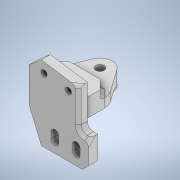
# Autodesk Inventor part: belt_holder_1
Saved by Autodesk Inventor 2020 (Build 240168000, 168)
## iProperties
Created: 2019-05-20
Part Number: belt_holder_1
Material: Generic
Document SubType Name: Modeling
Designer: psrob
Density: 1 g/cm^3
Appearance: Default
Author: psrob
Autodesk Inventor part; units mm, degrees
ref_plane "YZ Plane" through (0, 0, 0) normal (1, 0, 0) x (0, 1, 0)
ref_plane "XZ Plane" through (0, 0, 0) normal (0, 1, 0) x (-1, 0, 0)
ref_plane "XY Plane" through (0, 0, 0) normal (0, 0, 1) x (1, 0, 0)
sketch "Sketch1" plane through (0, 0, 0) normal (0, 0, 1) x (1, 0, 0)
  circle A0 centre (4.591147, -15.25) radius 1.5
  circle A1 centre (11.591147, -15.25) radius 1.5
  circle A2 centre (1.281, 33.75) radius 1
  circle A3 centre (9.281, 32.75) radius 1
  circle A4 centre (-9.854667, 17.759187) radius 1.5
  ellipse E0 centre (11.591147, 1.75) end of major axis (11.591147, 0.25) minor radius 1.5
  ellipse E1 centre (4.591147, 1.75) end of major axis (4.591147, 0.25) minor radius 1.5
  line L0 (15.854667, -21.335738) -> (15.854667, -7.75)
  line L1 (15.854667, -7.75) -> (15.854667, 31.319988)
  arc A5 (15.854667, 31.319988) -> (12.464791, 35.273183) centre (11.854667, 31.319988) ccw
  line L2 (12.464791, 35.273183) -> (-3.583333, 37.75)
  line L3 (-3.583333, 37.75) -> (-15.854667, 37.75)
  line L4 (-15.854667, 37.75) -> (-15.854667, 17.759187)
  arc A6 (-15.854667, 17.759187) -> (-12.464791, 13.805992) centre (-11.854667, 17.759187) ccw
  line L5 (-12.464791, 13.805992) -> (-4.228148, 12.534774)
  arc A7 (0.856667, 6.604982) -> (-4.228148, 12.534774) centre (-5.143333, 6.604982) ccw
  line L6 (0.856667, 6.604982) -> (0.856667, -10.595544)
  arc A8 (-2.560097, -18.122894) -> (0.856667, -10.595544) centre (-9.143333, -10.595544) ccw
  line L7 (-2.560097, -18.122894) -> (-15.854667, -29.75)
  line L8 (-15.854667, -29.75) -> (-15.854667, -37.75)
  line L9 (-15.854667, -37.75) -> (-3.583333, -37.75)
  line L10 (-3.583333, -37.75) -> (13.592861, -22.72812)
  arc A9 (15.854667, -21.335738) -> (13.592861, -22.72812) centre (18.85945, -28.75) ccw
  arc A10 (3.60693, 16.35) -> (6.10693, 16.35) centre (4.85693, 16.35) ccw
  line L11 (3.60693, 16.35) -> (3.60693, 18.35)
  arc A11 (6.10693, 18.35) -> (3.60693, 18.35) centre (4.85693, 18.35) ccw
  line L12 (6.10693, 18.35) -> (6.10693, 16.35)
  arc A12 (10.60934, 16.35) -> (13.10934, 16.35) centre (11.85934, 16.35) ccw
  line L13 (10.60934, 16.35) -> (10.60934, 18.35)
  arc A13 (13.10934, 18.35) -> (10.60934, 18.35) centre (11.85934, 18.35) ccw
  line L14 (13.10934, 18.35) -> (13.10934, 16.35)
  line L15 (-8.583333, 23.75) -> (-8.583333, 27.75)
  arc A14 (-6.583333, 29.75) -> (-8.583333, 27.75) centre (-6.583333, 27.75) ccw
  line L16 (-6.583333, 29.75) -> (9.854667, 29.75)
  arc A15 (11.854667, 27.75) -> (9.854667, 29.75) centre (9.854667, 27.75) ccw
  line L17 (11.854667, 27.75) -> (11.854667, 23.75)
  arc A16 (9.854667, 21.75) -> (11.854667, 23.75) centre (9.854667, 23.75) ccw
  line L18 (9.854667, 21.75) -> (-6.583333, 21.75)
  arc A17 (-8.583333, 23.75) -> (-6.583333, 21.75) centre (-6.583333, 23.75) ccw
  circle A18 centre (-12.719, 33.75) radius 1.5
  circle A19 centre (-6.719, 33.75) radius 1.5
  circle A20 centre (-6.719, -33.75) radius 1.5
  circle A21 centre (-12.719, -33.75) radius 1.5
  circle A22 centre (-9.854667, 17.759187) radius 1.5
  line L19 (-6.228148, 21.534774) -> (-4.228148, 19.534774)
  line L20 (-6.228148, 21.534774) -> (-17.275997, 21.534774)
  ellipse E2 centre (-17.275997, 27.534774) end of major axis (-8.634403, 27.534774) minor radius 6 (-21.607006, 22.342722) -> (-17.275997, 21.534774) ccw
  line L21 (-21.607006, 14.234289) -> (-21.607006, 22.342722)
  ellipse E3 centre (-20.359628, 10.329175) end of major axis (-26.120691, 10.329175) minor radius 4 (-20.359628, 14.329175) -> (-21.607006, 14.234289) ccw
  line L22 (-15.854667, 14.329175) -> (-20.359628, 14.329175)
  line L23 (-15.854667, 14.329175) -> (-7.193044, 12.992367)
  line L24 (-4.228148, 15.534774) -> (-7.193044, 12.992367)
  line L25 (-4.228148, 15.534774) -> (-4.228148, 19.534774)
  line L26 (-3.583333, 37.75) -> (-3.583333, 12.75)
  line L27 (-3.583333, 12.75) -> (15.854667, 12.75)
  line L28 (15.854667, 31.319988) -> (15.854667, 12.75)
  point P0 (0, 0)
  dimension "d0" = 25
  constraints: 6 end point, 1 collinear, 1 perpendicular, 1 point on line, 1 vertical, 2 other
  measures "d0" distance of L2.end L26.end
extrude "Extrusion1" add sketch "Sketch1" along normal blind 4 contours L27 L26 L18 A16 L17 A15 L16 L2 A5 L1 | L26 L16 A15 L17 A16 L18
sketch "Sketch2" plane through (0, 0, 0) normal (0, 0, -1) x (-1, 0, 0)
  line L0 (-9.854667, 29.75) -> (6.583333, 29.75)
  arc A0 (8.583333, 27.75) -> (6.583333, 29.75) centre (6.583333, 27.75) ccw
  line L1 (8.583333, 27.75) -> (8.583333, 23.75)
  circle A1 centre (-1.281, 33.75) radius 1
  circle A2 centre (-9.281, 32.75) radius 1
  circle A3 centre (9.854667, 17.759187) radius 1.5
  ellipse E0 centre (-11.591147, 1.75) end of major axis (-11.591147, 0.25) minor radius 1.5
  ellipse E1 centre (-4.591147, 1.75) end of major axis (-4.591147, 0.25) minor radius 1.5
  arc A4 (-6.10693, 16.35) -> (-3.60693, 16.35) centre (-4.85693, 16.35) ccw
  line L2 (-6.10693, 16.35) -> (-6.10693, 18.35)
  arc A5 (-3.60693, 18.35) -> (-6.10693, 18.35) centre (-4.85693, 18.35) ccw
  line L3 (-3.60693, 18.35) -> (-3.60693, 16.35)
  arc A6 (-13.10934, 16.35) -> (-10.60934, 16.35) centre (-11.85934, 16.35) ccw
  line L4 (-13.10934, 16.35) -> (-13.10934, 18.35)
  arc A7 (-10.60934, 18.35) -> (-13.10934, 18.35) centre (-11.85934, 18.35) ccw
  line L5 (-10.60934, 18.35) -> (-10.60934, 16.35)
  arc A8 (12.464791, 13.805992) -> (15.854667, 17.759187) centre (11.854667, 17.759187) ccw
  line L6 (15.854667, 17.759187) -> (15.854667, 37.75)
  line L7 (3.583333, 37.75) -> (15.854667, 37.75)
  line L8 (3.583333, 37.75) -> (-12.464791, 35.273183)
  arc A9 (-12.464791, 35.273183) -> (-15.854667, 31.319988) centre (-11.854667, 31.319988) ccw
  line L9 (-15.854667, 31.319988) -> (-15.854667, -3.75)
  line L10 (-0.856667, -3.75) -> (-15.854667, -3.75)
  line L11 (-0.856667, 6.604982) -> (-0.856667, -3.75)
  arc A10 (4.228148, 12.534774) -> (-0.856667, 6.604982) centre (5.143333, 6.604982) ccw
  line L12 (4.228148, 12.534774) -> (12.464791, 13.805992)
  circle A11 centre (6.719, 33.75) radius 1.5
  circle A12 centre (12.719, 33.75) radius 1.5
  line L13 (-9.854667, 29.75) -> (6.583333, 29.75)
  arc A13 (8.583333, 27.75) -> (6.583333, 29.75) centre (6.583333, 27.75) ccw
  line L14 (8.583333, 27.75) -> (8.583333, 23.75)
  arc A14 (6.583333, 21.75) -> (8.583333, 23.75) centre (6.583333, 23.75) ccw
  line L15 (6.583333, 21.75) -> (-9.854667, 21.75)
  arc A15 (-11.854667, 23.75) -> (-9.854667, 21.75) centre (-9.854667, 23.75) ccw
  line L16 (-11.854667, 23.75) -> (-11.854667, 27.75)
  arc A16 (-9.854667, 29.75) -> (-11.854667, 27.75) centre (-9.854667, 27.75) ccw
  line L17 (-9.854667, 27.75) -> (6.583333, 23.75)
  line L18 (6.583333, 23.75) -> (6.583333, 27.75)
  line L19 (6.583333, 27.75) -> (-9.854667, 23.75)
  line L20 (-9.635667, 28.25) -> (6.364333, 28.25)
  line L21 (6.364333, 28.25) -> (6.364333, 23.25)
  line L22 (6.364333, 23.25) -> (-9.635667, 23.25)
  line L23 (-9.635667, 23.25) -> (-9.635667, 28.25)
  line L24 (-9.635667, 28.25) -> (6.364333, 23.25) construction
  line L25 (6.364333, 28.25) -> (-9.635667, 23.25) construction
  point P0 (0, 0)
  point P1 (-1.635667, 25.75)
  dimension "d3" = 16
  dimension "d4" = 5
  constraints: 18 end point, 3 midpoint, 2 parallel, 1 horizontal, 1 perpendicular, 1 vertical, 2 other
  measures "d3" distance of L20.start L20.end
  measures "d4" distance of L20.end L21.end
extrude "Extrusion2" add sketch "Sketch2" along normal blind 10 contours L23 L20 L21 L19 L17 | L17 L19 L23 | L19 L21 L17 | L17 L21 L22 L23 L19
sketch "Sketch5" plane through (-6.364333, 28.25, 0) normal (0, 1, 0) x (1, 0, 0)
  line L0 (0, 0) -> (2.781, 0)
  line L1 (16, 0) -> (2.781, 0)
  line L2 (16, 0) -> (16, 10)
  line L3 (0, 10) -> (16, 10)
  line L4 (0, 0) -> (0, 10)
  circle A0 centre (21.963546, 21.566956) radius 5.35
  circle A1 centre (-9.490334, 18.594839) radius 3.75
  circle A2 centre (21.963546, 21.566956) radius 6
  circle A3 centre (-9.490334, 18.594839) radius 6
  line L5 (21.963546, 21.566956) -> (-9.490334, 18.594839)
  line L6 (6.236606, 20.080897) -> (6.42475, 18.089766)
  line L7 (6.42475, 18.089766) -> (1.944706, 17.666441)
  line L8 (1.944706, 17.666441) -> (10.904795, 18.513092)
  circle A4 centre (10.904795, 18.513092) radius 4.5
  circle A5 centre (1.944706, 17.666441) radius 4.5
  circle A6 centre (10.904795, 18.513092) radius 2.5
  circle A7 centre (1.944706, 17.666441) radius 2.5
  line L9 (10.904795, 18.513092) -> (10.669614, 21.002005)
  line L10 (10.669614, 21.002005) -> (1.709526, 20.155355)
  line L11 (1.944706, 17.666441) -> (1.709526, 20.155355)
  line L12 (16, 10) -> (13.393708, 18.748272)
  line L13 (0, 10) -> (-0.548603, 17.483665)
  line L14 (1.944706, 17.666441) -> (-0.548603, 17.483665)
  line L15 (10.904795, 18.513092) -> (13.393708, 18.748272)
  point P0 (6.364333, 0)
  dimension "d15" = 12
  dimension "d16" = 12
  dimension "d17" = 2
  dimension "d18" = 4.5
  dimension "d19" = 9
  dimension "d20" = 9
  dimension "d21" = 9
  dimension "d22" = 5
  dimension "d23" = 5
  constraints: 22 end point, 6 centre point, 6 coincident, 5 perpendicular, 4 point on circle, 3 point on line, 1 midpoint, 1 parallel
  measures "d15" diameter of A2
  measures "d16" diameter of A3
  measures "d17" distance of L6.start L6.end
  measures "d18" distance of L6.end L7.end
  measures "d19" distance of L7.end L8.end
  measures "d20" diameter of A4
  measures "d21" diameter of A5
  measures "d22" diameter of A6
  measures "d23" diameter of A7
extrude "Extrusion5" add sketch "Sketch5" against normal up to surface (5 mm away) contours L13 A5 A4 L12 L3 | L13 A7 L7 A5 | A4 L8 A6 L12 | L14 L7 A7 | A7 L5 L11 L14 | A5 L5 L6 | A4 L5 A6 L8 | L6 L5 A4 | L7 A7 L5 A5 | L15 L9 L5 A6 | A6 L8 L15 | A7 L11 L5 | L10 A4 L5 A5 | A5 L5 A7 L10 | L11 L5 A7 L7 | A6 L5 L9 L8 | A4 L10 A6 L5 | L5 L9 A6 | L11 A7 L5 | A6 L9 L5 picked at (3.816876, 20.111221) picked at (8.607828, 20.563924)
thicken "Thicken1" operation add thickness 1 both sides no extend neighbours yes toward (0, -1, 0) faces at (-0.104, 23.25, -6.666667)
sketch "Sketch6" plane through (-6.364333, 28.25, 0) normal (0, 1, 0) x (1, 0, 0)
  line L0 (0, 0) -> (2.781, 0)
  line L1 (16, 0) -> (2.781, 0)
  line L2 (16, 0) -> (16, 10)
  line L3 (16, 10) -> (13.393708, 18.748272)
  arc A0 (13.393708, 18.748272) -> (10.669614, 21.002005) centre (10.904795, 18.513092) ccw
  line L4 (10.669614, 21.002005) -> (1.709526, 20.155355)
  arc A1 (1.709526, 20.155355) -> (-0.548603, 17.483665) centre (1.944706, 17.666441) ccw
  line L5 (-0.548603, 17.483665) -> (0, 10)
  line L6 (0, 0) -> (0, 10)
  line L7 (10.904795, 18.513092) -> (1.944706, 17.666441)
  line L8 (31.878318, 14.46818) -> (-17.899951, 9.764568)
  line L9 (-17.899951, 9.764568) -> (-19.028817, 21.711353)
  line L10 (-19.028817, 21.711353) -> (30.749451, 26.414965)
  line L11 (30.749451, 26.414965) -> (31.878318, 14.46818)
  line L12 (31.878318, 14.46818) -> (-19.028817, 21.711353) construction
  line L13 (-17.899951, 9.764568) -> (30.749451, 26.414965) construction
  point P0 (6.364333, 0)
  point P1 (6.42475, 18.089766)
  dimension "d28" = 50
  dimension "d29" = 12
  constraints: 14 end point, 3 midpoint, 2 parallel, 1 perpendicular
  measures "d28" distance of L8.start L8.end
  measures "d29" distance of L8.end L9.end
extrude "Extrusion6" cut sketch "Sketch6" against normal blind 3 contours L8 L9 L10 L11 L3 A0 L4 A1 L5 | L5 A1 L4 A0 L3 L8
sketch "Sketch9" plane through (0, 0, 0) normal (0, 0, -1) x (-1, 0, 0)
  line L0 (-9.635667, 28.25) -> (3.583333, 28.25)
  line L1 (3.583333, 37.75) -> (3.583333, 28.25)
  line L2 (-12.464791, 35.273183) -> (3.583333, 37.75)
  arc A0 (-12.464791, 35.273183) -> (-15.854667, 31.319988) centre (-11.854667, 31.319988) ccw
  line L3 (-15.854667, 12.75) -> (-15.854667, 31.319988)
  line L4 (3.583333, 12.75) -> (-15.854667, 12.75)
  line L5 (3.583333, 22.25) -> (3.583333, 12.75)
  line L6 (3.583333, 22.25) -> (-9.635667, 22.25)
  line L7 (-9.635667, 22.25) -> (-9.635667, 28.25)
  circle A1 centre (-1.281, 33.75) radius 1
  circle A2 centre (-9.281, 32.75) radius 1
  arc A3 (-13.10934, 16.35) -> (-10.60934, 16.35) centre (-11.85934, 16.35) ccw
  line L8 (-13.10934, 18.35) -> (-13.10934, 16.35)
  arc A4 (-10.60934, 18.35) -> (-13.10934, 18.35) centre (-11.85934, 18.35) ccw
  line L9 (-10.60934, 16.35) -> (-10.60934, 18.35)
  arc A5 (-6.10693, 16.35) -> (-3.60693, 16.35) centre (-4.85693, 16.35) ccw
  line L10 (-6.10693, 18.35) -> (-6.10693, 16.35)
  arc A6 (-3.60693, 18.35) -> (-6.10693, 18.35) centre (-4.85693, 18.35) ccw
  line L11 (-3.60693, 16.35) -> (-3.60693, 18.35)
  arc A7 (-12.464791, 35.273183) -> (-15.854667, 31.319988) centre (-11.854667, 31.319988) ccw
  line L12 (-15.854667, 12.75) -> (-15.854667, 31.319988)
  line L13 (-12.464791, 35.273183) -> (-15.854667, 35.273183)
  line L14 (-15.854667, 35.273183) -> (-15.854667, 22.25)
  line L15 (-15.854667, 22.25) -> (-12.464791, 22.25)
  line L16 (-12.464791, 22.25) -> (-12.464791, 35.273183)
  point P0 (0, 0)
  point P1 (-15.854667, 31.319988)
  constraints: 8 end point, 2 parallel, 1 horizontal, 1 perpendicular, 1 point on line
extrude "Extrusion9" cut sketch "Sketch9" against normal blind 4 contours L16 L15 L3 A0 | A0 L14 L13
sketch "Sketch10" plane through (0, 0, 0) normal (0, 0, -1) x (-1, 0, 0)
  line L0 (-12.464791, 22.25) -> (-15.854667, 22.25)
  line L1 (-15.854667, 12.75) -> (-15.854667, 22.25)
  line L2 (3.583333, 12.75) -> (-15.854667, 12.75)
  line L3 (3.583333, 22.25) -> (3.583333, 12.75)
  line L4 (3.583333, 22.25) -> (-9.635667, 22.25)
  line L5 (-9.635667, 22.25) -> (-9.635667, 28.25)
  line L6 (-9.635667, 28.25) -> (3.583333, 28.25)
  line L7 (3.583333, 37.75) -> (3.583333, 28.25)
  line L8 (-12.464791, 35.273183) -> (3.583333, 37.75)
  line L9 (-12.464791, 35.273183) -> (-12.464791, 22.25)
  circle A0 centre (-1.281, 33.75) radius 1
  circle A1 centre (-9.281, 32.75) radius 1
  arc A2 (-13.10934, 16.35) -> (-10.60934, 16.35) centre (-11.85934, 16.35) ccw
  line L10 (-13.10934, 18.35) -> (-13.10934, 16.35)
  arc A3 (-10.60934, 18.35) -> (-13.10934, 18.35) centre (-11.85934, 18.35) ccw
  line L11 (-10.60934, 16.35) -> (-10.60934, 18.35)
  arc A4 (-6.10693, 16.35) -> (-3.60693, 16.35) centre (-4.85693, 16.35) ccw
  line L12 (-6.10693, 18.35) -> (-6.10693, 16.35)
  arc A5 (-3.60693, 18.35) -> (-6.10693, 18.35) centre (-4.85693, 18.35) ccw
  line L13 (-3.60693, 16.35) -> (-3.60693, 18.35)
  line L14 (3.583333, 12.75) -> (-15.854667, 12.75)
  line L15 (3.583333, 12.75) -> (-0.416667, 12.75)
  line L16 (-0.416667, 12.75) -> (-0.416667, 22.25)
  line L17 (-0.416667, 22.25) -> (3.583333, 22.25)
  line L18 (3.583333, 22.25) -> (3.583333, 12.75)
  point P0 (0, 0)
  dimension "d44" = 4
  dimension "d45" = 9.5
  constraints: 8 end point, 2 parallel, 1 horizontal, 1 perpendicular
  measures "d44" distance of L16.end L17.end
  measures "d45" distance of L15.end L16.end
extrude "Extrusion10" cut sketch "Sketch10" against normal blind 4 contours L16 L4 L3 L2
sketch "Sketch11" plane through (-6.364333, 22.25, 0) normal (0, -1, 0) x (1, 0, 0)
  line L0 (16, -10) -> (13.393708, -18.748272)
  line L1 (16, 0) -> (16, -10)
  line L2 (6.781, 0) -> (16, 0)
  line L3 (6.781, 0) -> (6.781, 4)
  line L4 (2.781, 4) -> (6.781, 4)
  line L5 (2.781, 0) -> (2.781, 4)
  line L6 (2.781, 0) -> (0, 0)
  line L7 (0, 0) -> (0, -10)
  line L8 (-0.548603, -17.483665) -> (0, -10)
  line L9 (10.669614, -21.002005) -> (1.709526, -20.155355)
  line L10 (0, 0) -> (0, -4)
  line L11 (0, 0) -> (0, -10)
  line L12 (0, -4) -> (2.781, 0)
  arc A0 (-0.548603, -17.483665) -> (1.709526, -20.155355) centre (1.944706, -17.666441) ccw
  arc A1 (10.669614, -21.002005) -> (13.393708, -18.748272) centre (10.904795, -18.513092) ccw
  point P0 (6.364333, 0)
  dimension "d48" = 4
  constraints: 4 end point, 1 point on line
  measures "d48" distance of L6.end L10.end
extrude "Extrusion11" cut sketch "Sketch11" against normal blind 6 contours L12 L7 L6
sketch "Sketch12" plane through (9.635667, 28.25, 0) normal (0, 1, 0) x (1, 0, 0)
  line L0 (-16, 4) -> (-13.219, 0)
  line L1 (0, 0) -> (-13.219, 0)
  line L2 (0, 0) -> (0, 10)
  line L3 (0, 10) -> (-0.859966, 12.886558)
  line L4 (-0.859966, 12.886558) -> (-16.105997, 11.445942)
  line L5 (-16.105997, 11.445942) -> (-16, 10)
  line L6 (-16, 4) -> (-16, 10)
  line L7 (-16.105997, 11.445942) -> (-13.119301, 11.728158)
  line L8 (-0.859966, 12.886558) -> (-16.105997, 11.445942)
  line L9 (-13.119301, 11.728158) -> (-16, 10)
  line L10 (-0.859966, 12.886558) -> (-3.846662, 12.604342)
  line L11 (-3.846662, 12.604342) -> (0, 10)
  point P0 (-9.635667, 0)
  dimension "d51" = 3
  dimension "d52" = 3
  constraints: 8 end point, 2 point on line
  measures "d51" distance of L4.end L7.end
  measures "d52" distance of L3.end L10.end
extrude "Extrusion12" cut sketch "Sketch12" against normal up to surface (3 mm away) contours L5 L4 L9 | L11 L4 L3
sketch "Sketch13" plane through (0, 0, 4) normal (0, 0, 1) x (1, 0, 0)
  line L0 (0.416667, 22.25) -> (0.416667, 12.75)
  line L1 (0.416667, 12.75) -> (15.854667, 12.75)
  line L2 (15.854667, 12.75) -> (15.854667, 22.25)
  line L3 (15.854667, 22.25) -> (12.464791, 22.25)
  line L4 (12.464791, 22.25) -> (12.464791, 35.273183)
  line L5 (12.464791, 35.273183) -> (-3.583333, 37.75)
  line L6 (-3.583333, 37.75) -> (-3.583333, 22.25)
  line L7 (-3.583333, 22.25) -> (0.416667, 22.25)
  circle A0 centre (1.281, 33.75) radius 1
  circle A1 centre (9.281, 32.75) radius 1
  arc A2 (10.60934, 16.35) -> (13.10934, 16.35) centre (11.85934, 16.35) ccw
  line L8 (10.60934, 16.35) -> (10.60934, 18.35)
  arc A3 (13.10934, 18.35) -> (10.60934, 18.35) centre (11.85934, 18.35) ccw
  line L9 (13.10934, 18.35) -> (13.10934, 16.35)
  arc A4 (3.60693, 16.35) -> (6.10693, 16.35) centre (4.85693, 16.35) ccw
  line L10 (3.60693, 16.35) -> (3.60693, 18.35)
  arc A5 (6.10693, 18.35) -> (3.60693, 18.35) centre (4.85693, 18.35) ccw
  line L11 (6.10693, 18.35) -> (6.10693, 16.35)
  line L12 (-3.583333, 28.25) -> (-3.583333, 22.25)
  line L13 (0.416667, 12.75) -> (-3.583333, 22.25)
  point P0 (0, 0)
  point P1 (-3.583333, 29.25)
  constraints: 2 end point
extrude "Extrusion13" add sketch "Sketch13" against normal blind 4 contours L0 L13 L7
chamfer "Chamfer1" distance 4 angle 45 1 edges at (-3.5833, 37.75, 2)
thicken "Thicken2" operation add thickness 1 both sides no extend neighbours yes toward (0, 0, -1) faces at (0.743959, 24.84202, 4)
fillet "Fillet5" radius 2 1 edges at (12.4648, 22.25, 1.5)
chamfer "Chamfer3" distance 1 angle 45 3 edges at (13.0506, 22.8358, 3) (15.1597, 22.25, 3) (12.4648, 29.7616, 3)
chamfer "Chamfer4" distance 2 angle 45 1 edges at (15.8547, 12.75, 1.5)
fillet "Fillet6" radius 1 2 edges at (15.8547, 21.75, 2.5) (11.9648, 35.3504, 2.5)
sketch "Sketch17" plane through (-6.364333, 25.25, 0) normal (0, 1, 0) x (1, 0, 0)
  line L0 (13.393708, 18.748272) -> (16, 10)
  arc A0 (13.393708, 18.748272) -> (10.669614, 21.002005) centre (10.904795, 18.513092) ccw
  line L1 (1.709526, 20.155355) -> (10.669614, 21.002005)
  arc A1 (1.709526, 20.155355) -> (-0.548603, 17.483665) centre (1.944706, 17.666441) ccw
  line L2 (0, 10) -> (-0.548603, 17.483665)
  line L3 (-0.122828, 11.67553) -> (-0.548603, 17.483665)
  line L4 (13.393708, 18.748272) -> (-0.548603, 17.483665)
  line L5 (0, 10) -> (2.880699, 11.728158)
  line L6 (12.153338, 12.604342) -> (2.880699, 11.728158)
  line L7 (12.153338, 12.604342) -> (16, 10)
  point P0 (6.364333, 0)
  constraints: 2 end point
extrude "Extrusion17" cut sketch "Sketch17" against normal blind 10 contours L4 A1 L1 A0
sketch "Sketch18" plane through (-6.364333, 25.25, 0) normal (0, 1, 0) x (1, 0, 0)
  line L0 (13.393708, 18.748272) -> (-0.548603, 17.483665)
  line L1 (0, 10) -> (-0.548603, 17.483665)
  line L2 (13.393708, 18.748272) -> (16, 10)
  line L3 (13.393708, 18.748272) -> (13.964746, 16.831526)
  line L4 (13.393708, 18.748272) -> (15.323973, 12.269149)
  line L5 (13.964746, 16.831526) -> (-0.405249, 15.528127)
  line L6 (-0.548603, 17.483665) -> (0, 10)
  line L7 (13.393708, 18.748272) -> (-0.548603, 17.483665)
  line L8 (-0.405249, 15.528127) -> (-0.548603, 17.483665)
  line L9 (0, 10) -> (2.880699, 11.728158)
  line L10 (12.153338, 12.604342) -> (2.880699, 11.728158)
  line L11 (12.153338, 12.604342) -> (16, 10)
  point P0 (6.364333, 0)
  point P1 (-0.122828, 11.67553)
  point P2 (-0.405249, 15.528127)
  dimension "d108" = 2
  constraints: 6 end point, 2 point on line, 1 collinear, 1 parallel
  measures "d108" distance of L0.start L3.end
extrude "Extrusion23" cut sketch "Sketch18" against normal blind 10 contours L2 L5 L1 L0
sketch "Sketch23" plane through (-3.583333, 28.25, 0) normal (0, 1, 0) x (1, 0, 0)
  line L0 (0.099699, 11.728158) -> (-2.781, 10)
  line L1 (-2.781, 4) -> (-2.781, 10)
  line L2 (-2.781, 4) -> (0, 0)
  line L3 (13.219, 0) -> (0, 0)
  line L4 (13.219, 0) -> (13.219, 10)
  line L5 (13.219, 10) -> (9.372338, 12.604342)
  line L6 (9.372338, 12.604342) -> (0.099699, 11.728158)
  line L7 (13.219, 10) -> (9.372338, 12.604342)
  line L8 (13.219, 10) -> (-2.781, 10)
  point P0 (3.583333, 0)
  constraints: 2 end point, 1 horizontal
extrude "Extrusion24" cut sketch "Sketch23" against normal up to surface (3 mm away) contours L6 L5 L8 L0
sketch "Sketch24" plane through (-6.364333, 25.25, 0) normal (0, 1, 0) x (1, 0, 0)
  line L0 (13.964746, 16.831526) -> (-0.405249, 15.528127)
  line L1 (0, 10) -> (-0.405249, 15.528127)
  line L2 (0, 10) -> (16, 10)
  line L3 (13.964746, 16.831526) -> (16, 10)
  line L4 (13.964746, 16.831526) -> (-0.405249, 15.528127)
  circle A0 centre (6.779749, 16.179826) radius 4
  line L5 (6.779749, 16.179826) -> (10.054542, 18.476722)
  line L6 (6.779749, 16.179826) -> (3.065789, 17.665258)
  line L7 (0, 10) -> (-0.405249, 15.528127)
  line L8 (3.065789, 17.665258) -> (0, 10)
  line L9 (16, 0) -> (16, 10)
  line L10 (10.054542, 18.476722) -> (16, 10)
  arc A1 (10.054542, 18.476722) -> (3.065789, 17.665258) centre (6.779749, 16.179826) ccw
  line L11 (13.964746, 16.831526) -> (-0.405249, 15.528127)
  line L12 (0, 10) -> (-0.405249, 15.528127)
  line L13 (0, 10) -> (16, 10)
  line L14 (13.964746, 16.831526) -> (16, 10)
  line L15 (13.964746, 16.831526) -> (-0.405249, 15.528127)
  circle A2 centre (6.779749, 16.179826) radius 4
  line L16 (6.779749, 16.179826) -> (10.054542, 18.476722)
  line L17 (6.779749, 16.179826) -> (3.065789, 17.665258)
  line L18 (0, 10) -> (-0.405249, 15.528127)
  line L19 (3.065789, 17.665258) -> (0, 10)
  line L20 (16, 0) -> (16, 10)
  line L21 (10.054542, 18.476722) -> (16, 10)
  arc A3 (10.054542, 18.476722) -> (3.065789, 17.665258) centre (6.779749, 16.179826) ccw
  point P0 (6.364333, 0)
  point P1 (6.364333, 0)
  point P2 (2.309509, 15.774363)
  point P3 (11.373321, 16.596476)
  dimension "d113" = 8
  dimension "d114" = 4
  dimension "d115" = 8
  dimension "d116" = 4
  constraints: 30 end point, 8 point on circle, 4 centre point, 4 perpendicular, 2 midpoint
  measures "d113" diameter of A0
  measures "d114" radius of A1
  measures "d115" diameter of A2
  measures "d116" radius of A3
sketch "Sketch25" plane through (-6.364333, 25.25, 0) normal (0, 1, 0) x (1, 0, 0)
  line L0 (13.964746, 16.831526) -> (-0.405249, 15.528127)
  line L1 (0, 10) -> (-0.405249, 15.528127)
  line L2 (0, 10) -> (16, 10)
  line L3 (13.964746, 16.831526) -> (16, 10)
  line L4 (13.964746, 16.831526) -> (-0.405249, 15.528127)
  circle A0 centre (6.779749, 16.179826) radius 4
  line L5 (6.779749, 16.179826) -> (10.054542, 18.476722)
  line L6 (6.779749, 16.179826) -> (3.065789, 17.665258)
  line L7 (0, 10) -> (-0.405249, 15.528127)
  line L8 (3.065789, 17.665258) -> (0, 10)
  line L9 (16, 0) -> (16, 10)
  line L10 (10.054542, 18.476722) -> (16, 10)
  arc A1 (10.054542, 18.476722) -> (3.065789, 17.665258) centre (6.779749, 16.179826) ccw
  line L11 (13.964746, 16.831526) -> (-0.405249, 15.528127)
  line L12 (0, 10) -> (-0.405249, 15.528127)
  line L13 (0, 10) -> (16, 10)
  line L14 (13.964746, 16.831526) -> (16, 10)
  line L15 (13.964746, 16.831526) -> (-0.405249, 15.528127)
  circle A2 centre (6.779749, 16.179826) radius 4
  line L16 (6.779749, 16.179826) -> (10.054542, 18.476722)
  line L17 (6.779749, 16.179826) -> (3.065789, 17.665258)
  line L18 (0, 10) -> (-0.405249, 15.528127)
  line L19 (3.065789, 17.665258) -> (0, 10)
  line L20 (16, 0) -> (16, 10)
  line L21 (10.054542, 18.476722) -> (16, 10)
  arc A3 (10.054542, 18.476722) -> (3.065789, 17.665258) centre (6.779749, 16.179826) ccw
  point P0 (6.364333, 0)
  point P1 (6.364333, 0)
  point P2 (6.364333, 0)
  point P3 (11.373321, 16.596476)
  point P4 (2.309509, 15.774363)
  dimension "d117" = 8
  dimension "d118" = 4
  dimension "d119" = 8
  dimension "d120" = 4
  constraints: 44 end point, 8 point on circle, 4 centre point, 4 perpendicular, 2 midpoint
  measures "d117" diameter of A0
  measures "d118" radius of A1
  measures "d119" diameter of A2
  measures "d120" radius of A3
extrude "Extrusion25" cut sketch "Sketch24" against normal blind 10 contours L3 L10 L0 | L1 L0 L8
extrude "Extrusion26" add sketch "Sketch25" against normal up to surface (3 mm away) contours L0 A0 L10 | L0 L5 A0 | L5 L6 A0 | L0 A0 L6 | A0 L0 L8
sketch "Sketch26" plane through (-3.583333, 22.25, 0) normal (0, -1, 0) x (1, 0, 0)
  line L0 (0.284789, -17.665258) -> (-2.781, -10)
  arc A0 (0.284789, -17.665258) -> (7.273542, -18.476722) centre (3.998749, -16.179826) ccw
  line L1 (7.273542, -18.476722) -> (13.219, -10)
  line L2 (13.219, 0) -> (13.219, -10)
  line L3 (0, 0) -> (13.219, 0)
  line L4 (0, 0) -> (-2.781, -4)
  line L5 (-2.781, -4) -> (-2.781, -10)
  circle A1 centre (3.998749, -16.179826) radius 4
  point P0 (3.583333, 0)
  point P1 (7.273542, -18.476722)
  dimension "d125" = 8
  constraints: 1 centre point, 1 coincident
  measures "d125" diameter of A1
extrude "Extrusion27" add sketch "Sketch26" along normal blind 2 contours A1 A0
fillet "Fillet9" radius 2 1 edges at (0.8768, 22.25, -12.2065)
sketch "Sketch27" plane through (-3.583333, 20.25, 0) normal (0, -1, 0) x (1, 0, 0)
  arc A0 (7.273542, -18.476722) -> (0.284789, -17.665258) centre (3.998749, -16.179826) ccw
  arc A1 (0.284789, -17.665258) -> (7.273542, -18.476722) centre (3.998749, -16.179826) ccw
  circle A2 centre (3.998749, -16.179826) radius 1.4
  point P0 (3.583333, 0)
  dimension "d129" = 2.8
  constraints: 1 centre point, 1 coincident
  measures "d129" diameter of A2
extrude "Extrusion28" cut sketch "Sketch27" against normal blind 10 contours A2
chamfer "Chamfer5" distance 3 angle 45 2 edges at (-6.3643, 26.75, -10) (9.6357, 26.75, -10)
fillet "Fillet10" radius 1 3 edges at (-4.8643, 25.25, -8.5) (1.6357, 25.25, -10) (8.1357, 25.25, -8.5)
fillet "Fillet11" radius 5 2 edges at (-6.3643, 23.75, -10) (9.6357, 23.75, -10)
body "Solid1"
